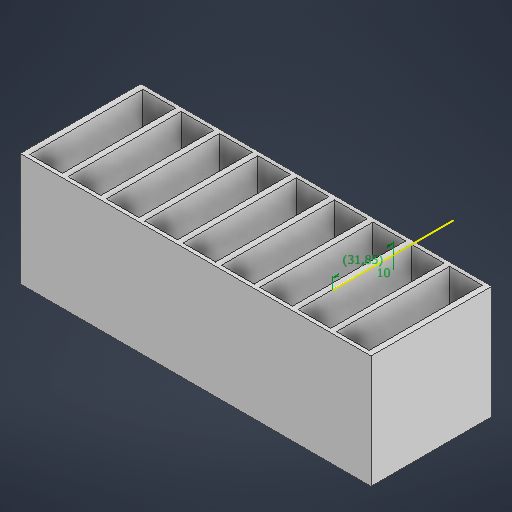
# Autodesk Inventor part: Base_Principal
Saved by Autodesk Inventor 2026 (Build 300175000, 175)
## iProperties
Created: 2025-04-04
Part Number: Base_Principal
Material: Genérico
Document SubType Name: Modeling
Designer: LabB305
Density: 1 g/cm^3
Appearance: Valor por defecto
Author: LabB305
Autodesk Inventor part; units mm, degrees
ref_plane "YZ Plane" through (0, 0, 0) normal (1, 0, 0) x (0, 1, 0)
ref_plane "XZ Plane" through (0, 0, 0) normal (0, 1, 0) x (-1, 0, 0)
ref_plane "XY Plane" through (0, 0, 0) normal (0, 0, 1) x (1, 0, 0)
sketch "Boceto1" plane through (0, 0, 0) normal (0, 1, 0) x (-1, 0, 0)
  line L0 (0, 0) -> (100, 0)
  line L1 (100, 0) -> (100, -31.85)
  line L2 (100, -31.85) -> (-100, -31.85)
  line L3 (-100, -31.85) -> (-100, 31.85)
  line L4 (-100, 31.85) -> (100, 31.85)
  line L5 (100, 31.85) -> (100, -31.85)
  dimension "d0" = 100
  dimension "d1" = 31.85
  dimension "d2" = 200
  dimension "d3" = 63.7
  constraints: 12 end point, 2 horizontal, 2 parallel, 2 perpendicular
  measures "d0" distance of L0.start L0.end
  measures "d1" distance of L0.end L1.end
  measures "d2" distance of L3.end L4.end
  measures "d3" distance of L2.end L3.end
extrude "Extrusión1" add sketch "Boceto1" along normal blind 76.62
sketch "Boceto2" plane through (0, 76.62, 0) normal (0, 1, 0) x (1, 0, 0)
  line L0 (-100, 31.85) -> (-100, -31.85) projected
  line L1 (-100, 0) -> (-97, 0)
  line L2 (-97, 0) -> (-97, 29.85)
  line L3 (-97, 29.85) -> (-79.76, 29.85)
  line L4 (-97, 29.85) -> (-79.76, 29.85)
  line L5 (-79.76, 29.85) -> (-79.76, -29.85)
  line L6 (-79.76, -29.85) -> (-97, -29.85)
  line L7 (-97, -29.85) -> (-97, 29.85)
  line L8 (-79.76, 0) -> (-76.76, 0)
  line L9 (-76.76, 0) -> (-76.76, 29.85)
  line L10 (-76.76, 29.85) -> (-59.52, 29.85)
  line L11 (-59.52, 29.85) -> (-59.52, -29.85)
  line L12 (-59.52, -29.85) -> (-76.76, -29.85)
  line L13 (-76.76, -29.85) -> (-76.76, 29.85)
  line L14 (-59.52, 0) -> (-56.52, 0)
  line L15 (-56.52, 0) -> (-56.52, 29.85)
  line L16 (-56.52, 29.85) -> (-39.28, 29.85)
  line L17 (-39.28, 29.85) -> (-39.28, -29.85)
  line L18 (-39.28, -29.85) -> (-56.52, -29.85)
  line L19 (-56.52, -29.85) -> (-56.52, 29.85)
  line L20 (-39.28, 0) -> (-36.28, 0)
  line L21 (-36.28, 0) -> (-36.28, 29.85)
  line L22 (-36.28, 29.85) -> (-19.04, 29.85)
  line L23 (-19.04, 29.85) -> (-19.04, -29.85)
  line L24 (-19.04, -29.85) -> (-36.28, -29.85)
  line L25 (-36.28, -29.85) -> (-36.28, 29.85)
  line L26 (-19.04, 0) -> (-16.04, 0)
  line L27 (-16.04, 0) -> (-16.04, 29.85)
  line L28 (-16.04, 29.85) -> (1.2, 29.85)
  line L29 (1.2, 29.85) -> (1.2, -29.85)
  line L30 (1.2, -29.85) -> (-16.04, -29.85)
  line L31 (-16.04, -29.85) -> (-16.04, 29.85)
  line L32 (1.2, 0) -> (2.7, 0)
  line L33 (2.7, 0) -> (2.7, 9.0784)
  line L34 (82.16, 0) -> (82.16, 29.85)
  line L35 (82.16, 29.85) -> (64.92, 29.85)
  line L36 (64.92, 29.85) -> (64.92, -29.85)
  line L37 (64.92, -29.85) -> (82.16, -29.85)
  line L38 (82.16, -29.85) -> (82.16, 29.85)
  line L39 (64.92, 0) -> (61.92, 0)
  line L40 (61.92, 0) -> (61.92, 29.85)
  line L41 (61.92, 29.85) -> (44.68, 29.85)
  line L42 (44.68, 29.85) -> (44.68, -29.85)
  line L43 (44.68, -29.85) -> (61.92, -29.85)
  line L44 (61.92, -29.85) -> (61.92, 29.85)
  line L45 (44.68, 0) -> (41.68, 0)
  line L46 (41.68, 0) -> (41.68, 29.85)
  line L47 (41.68, 29.85) -> (24.44, 29.85)
  line L48 (24.44, 29.85) -> (24.44, -29.85)
  line L49 (24.44, -29.85) -> (41.68, -29.85)
  line L50 (41.68, -29.85) -> (41.68, 29.85)
  line L51 (24.44, 0) -> (21.44, 0)
  line L52 (21.44, 0) -> (21.44, 29.85)
  line L53 (21.44, 29.85) -> (4.2, 29.85)
  line L54 (4.2, 29.85) -> (4.2, -29.85)
  line L55 (4.2, -29.85) -> (21.44, -29.85)
  line L56 (21.44, -29.85) -> (21.44, 29.85)
  line L57 (82.16, 0) -> (85.16, 0)
  line L58 (85.16, 0) -> (85.16, 31.85)
  line L59 (100, -31.85) -> (100, 31.85) projected
  line L60 (85.16, 31.85) -> (100, 31.85)
  line L61 (100, 31.85) -> (100, -31.85)
  line L62 (100, -31.85) -> (85.16, -31.85)
  line L63 (85.16, -31.85) -> (85.16, 31.85)
  point P0 (0, 0)
  point P1 (5.4, 0)
  point P2 (4.2, 0)
  dimension "d6" = 3
  dimension "d7" = 29.85
  dimension "d8" = 17.24
  dimension "d9" = 17.24
  dimension "d10" = 59.7
  dimension "d11" = 3
  dimension "d12" = 17.24
  dimension "d13" = 59.7
  dimension "d14" = 3
  dimension "d15" = 17.24
  dimension "d16" = 59.7
  dimension "d17" = 3
  dimension "d18" = 17.24
  dimension "d19" = 59.7
  dimension "d20" = 3
  dimension "d21" = 17.24
  dimension "d22" = 59.7
  dimension "d23" = 1.5
  dimension "d24" = 3
  constraints: 124 end point, 25 symmetric about line, 14 perpendicular, 13 horizontal, 12 parallel, 6 midpoint, 2 point on line
  measures "d6" distance of L1.start L1.end
  measures "d7" distance of L1.end L2.end
  measures "d8" distance of L2.end L3.end
  measures "d9" distance of L5.end L6.end
  measures "d10" distance of L4.end L5.end
  measures "d11" distance of L8.start L8.end
  measures "d12" distance of L11.end L12.end
  measures "d13" distance of L10.end L11.end
  measures "d14" distance of L14.start L14.end
  measures "d15" distance of L17.end L18.end
  measures "d16" distance of L16.end L17.end
  measures "d17" distance of L20.start L20.end
  measures "d18" distance of L23.end L24.end
  measures "d19" distance of L22.end L23.end
  measures "d20" distance of L26.start L26.end
  measures "d21" distance of L29.end L30.end
  measures "d22" distance of L28.end L29.end
  measures "d23" distance of L32.start L32.end
  measures "d24" distance of L34.start L57.end
extrude "Extrusión2" cut sketch "Boceto2" against normal blind 76.62
sketch "Boceto3" plane through (64.92, 76.62, 29.85) normal (1, 0, 0) x (0, 0, -1)
  line L0 (-2, 0) -> (61.7, 0) projected
  line L1 (-2, 0) -> (29.85, 0)
  line L2 (29.85, 0) -> (19.85, 0)
  point P0 (29.85, -76.62)
  dimension "d27" = 31.85
  dimension "d28" = 10
  constraints: 4 end point, 1 midpoint, 1 point on line
  measures "d27" distance of L0.start L1.end
  measures "d28" distance of L1.end L2.end
sketch "Boceto4" plane through (0, 0, 0) normal (0, -1, 0) x (1, 0, 0)
  line L0 (-100, -31.85) -> (-100, 31.85) projected
  line L1 (-100, 31.85) -> (85.16, 31.85)
  line L2 (85.16, 31.85) -> (85.16, -31.85)
  line L3 (85.16, -31.85) -> (-100, -31.85)
  line L4 (-100, -31.85) -> (-100, 31.85)
  point P0 (0, 0)
  constraints: 8 end point, 2 parallel, 1 horizontal, 1 perpendicular
extrude "Extrusión3" add sketch "Boceto4" along normal blind 3
sketch "Boceto5" plane through (0, 76.62, 0) normal (0, 1, 0) x (1, 0, 0)
  line L0 (85.16, -31.85) -> (85.16, 31.85) projected
  line L1 (-100, -31.85) -> (85.16, -31.85)
  line L2 (85.16, -31.85) -> (85.16, 31.85)
  line L3 (85.16, 31.85) -> (-100, 31.85)
  line L4 (-100, 31.85) -> (-100, -31.85)
  point P0 (0, 0)
  constraints: 8 end point, 2 parallel, 1 horizontal, 1 perpendicular
extrude "Extrusión4" cut sketch "Boceto5" against normal blind 20
sketch "Boceto6" plane through (85.16, -3, -31.85) normal (0, 0, -1) x (-1, 0, 0)
  point P0 (85.16, 3)
equation "\"d3\" = 2 * d1"
equation "\"d9\" = d8"
equation "\"d10\" = 2 * d7"
equation "\"d12\" = d8"
equation "\"d13\" = 2 * d7"
equation "\"d15\" = d8"
equation "\"d16\" = 2 * d7"
equation "\"d18\" = d8"
equation "\"d19\" = 2 * d7"
equation "\"d21\" = d8"
equation "\"d22\" = 2 * d7"
